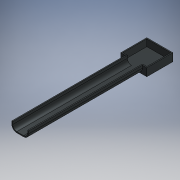
# Autodesk Inventor part: 手把A
Saved by Autodesk Inventor 2017 (Build 210142000, 142)
## iProperties
Part Number: 手把A
Material: SS41
Document SubType Name: Modeling
Designer: G
Density: 7.85 g/cm^3
Appearance: 鐵灰色
Author: G
Autodesk Inventor part; units mm, degrees
ref_plane "YZ Plane" through (0, 0, 0) normal (1, 0, 0) x (0, 1, 0)
ref_plane "XZ Plane" through (0, 0, 0) normal (0, 1, 0) x (-1, 0, 0)
ref_plane "XY Plane" through (0, 0, 0) normal (0, 0, 1) x (1, 0, 0)
sketch "草圖1" plane through (0, 0, 0) normal (0, 1, 0) x (-1, 0, 0)
  line L0 (-533.8511, -15) -> (-546.8433, -15)
  arc A0 (-556.8413, -5.002) -> (-546.8433, -15) centre (-546.8433, -5.002) ccw
  line L1 (-556.8413, -5.002) -> (-556.8413, -0.0001)
  arc A1 (-533.8511, -15) -> (-524.1171, -4.9412) centre (-534.1219, -4.9987) ccw
  line L2 (-524.1171, 0) -> (-524.1171, -4.9412)
  line L3 (-526.1171, 0) -> (-526.1171, -4.9473)
  arc A2 (-533.8796, -13) -> (-526.1171, -4.9473) centre (-534.1219, -4.9987) ccw
  line L4 (-533.8796, -13) -> (-546.8433, -13)
  arc A3 (-554.8413, -5.002) -> (-546.8433, -13) centre (-546.8433, -5.002) ccw
  line L5 (-554.8413, -5.002) -> (-554.8413, -0.0001)
  line L6 (-524.1171, 0) -> (-526.1171, 0)
  line L7 (-554.8413, -0.0001) -> (-556.8413, -0.0001)
  point P0 (0, 0)
  dimension "d0" = 2
  constraints: 16 end point, 8 point on circle, 4 centre point, 2 tangent, 1 horizontal, 1 parallel, 4 other
  measures "d0" distance between parallel lines of L2 L3
extrude "擠出1" add sketch "草圖1" along normal mid plane 218
sketch "草圖2" plane through (556.8413, -109, -0.0001) normal (0, 0, 1) x (1, 0, 0)
  line L0 (-41.4798, 268) -> (8.5202, 268)
  line L1 (8.5202, 268) -> (8.5202, 218)
  line L2 (8.5202, 218) -> (-41.4798, 218)
  line L3 (-41.4798, 218) -> (-41.4798, 268)
  line L4 (-22.9617, 218) -> (-9.998, 218) projected
  point P0 (-556.8413, 109)
  point P1 (-16.4798, 218)
  dimension "d3" = 50
  dimension "d4" = 50
  constraints: 8 end point, 2 midpoint, 2 parallel, 1 horizontal, 1 perpendicular
  measures "d3" distance of L1.end L2.end
  measures "d4" distance of L0.end L1.end
extrude "擠出2" add sketch "草圖2" against normal up to surface (14.9999 mm away) separate body
shell "薄殼1" thickness 2 removed faces 1 at (540.3615, 142.3333, -0.0001) bodies 2
combine bodies "合併1" operation type add bodies to combine 1 2
sketch "草圖3" plane through (515.3615, 109, -0.0001) normal (0, -1, 0) x (1, 0, 0)
  line L0 (10.7557, -4.9472) -> (10.7557, 0.0001) projected
  arc A0 (10.7557, -4.9472) -> (18.5182, -12.9999) centre (18.7605, -4.9986) ccw projected
  line L1 (31.4818, -12.9999) -> (18.5182, -12.9999) projected
  arc A1 (31.4818, -12.9999) -> (39.4798, -5.0019) centre (31.4818, -5.0019) ccw projected
  line L2 (39.4798, 0) -> (39.4798, -5.0019) projected
  line L3 (10.7557, 0.0001) -> (39.4798, 0)
  point P0 (-515.3615, 0.0001)
  constraints: 2 end point
extrude "擠出3" cut sketch "草圖3" against normal up to surface (2 mm away) bodies 1
move or copy body "移動本體1" bodies to move or copy 1 copy no translate (-540, 0, 0)
